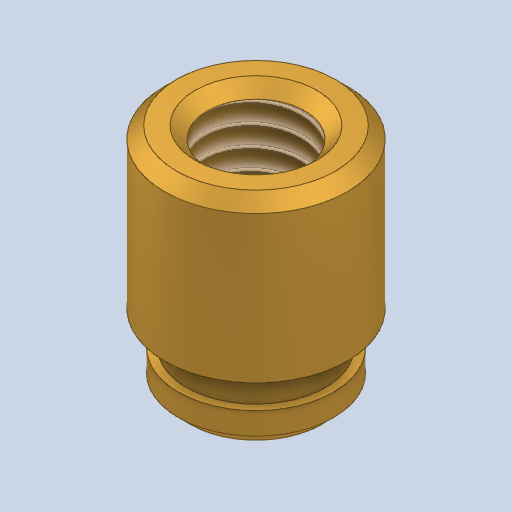
# Autodesk Inventor part: RX-M3x5,7
Saved by Autodesk Inventor 2023 (Build 270158000, 158)
## iProperties
Company: Ruthex
Created: 2022-06-20
Part Number: RX-M3x5,7
Material: Messing, weicher Gelbton
Document SubType Name: Modeling
Designer: buchmannmartin
Density: 8.47 g/cm^3
Appearance: Messing - satiniert
Description: RUTHEX Gewindeeinsatz-M3
Mass: 0.472484 g
Surface Area: 1.42553 cm^2
Volume: 0.0557832 cm^3
Author: buchmannmartin
Autodesk Inventor part; units mm, degrees
ref_plane "YZ Plane" through (0, 0, 0) normal (1, 0, 0) x (0, 1, 0)
ref_plane "XZ Plane" through (0, 0, 0) normal (0, 1, 0) x (-1, 0, 0)
ref_plane "XY Plane" through (0, 0, 0) normal (0, 0, 1) x (1, 0, 0)
sketch "Skizze1" plane through (0, 0, 0) normal (0, 0, 1) x (1, 0, 0)
  line L0 (0, 0) -> (0, 5.7)
  line L1 (0, 5.7) -> (-2.3, 5.7)
  line L2 (-2.3, 5.7) -> (-2.3, 1.71)
  line L3 (-2.3, 1.71) -> (-1.75, 1.71)
  line L4 (-1.75, 1.71) -> (-1.75, 0.855)
  line L5 (-1.75, 0.855) -> (-1.95, 0.855)
  line L6 (-1.95, 0.855) -> (-1.95, 0)
  line L7 (-1.95, 0) -> (0, 0)
  dimension "d0" = 4.6
  dimension "d1" = 5.7
  dimension "d2" = 3.9
  dimension "d3" = 0.2
  dimension "d4" = 3.99
  constraints: 16 end point, 7 perpendicular, 1 coincident, 1 parallel, 1 vertical
  measures "d0" diameter of L2 L0
  measures "d1" distance of L0.start L0.end
  measures "d2" diameter of L6 L0
  measures "d3" distance between parallel lines of L6 L4
  measures "d4" distance of L1.end L2.end
revolve "Umdrehung1" add sketch "Skizze1" angle 360 about axis through (0, 0, 0) along (0, 1, 0)
sketch "Skizze2" plane through (0, 5.7, 0) normal (0, 1, 0) x (1, 0, 0)
  circle A0 centre (0, 0) radius 2.3 projected
  constraints: 1 coincident
hole "Bohrung1" at (0, 5.7, 0) direction (0, -1, 0) diameter 2.459 end through all thread size "M3x0.5" class "6H" standard "ISO Metric profile"
chamfer "Fase1" distance 0.3 angle 45 4 edges at (0, 5.7, -1.2295) (1.95, 0, 0) (0, 0, -1.2295) (2.3, 5.7, 0)
equation "\"d4\" = 0.7 * d1"
